Autodesk Fusion 360 part; units mm, degrees
(part 3 of 6)
  spline S106 degree 5 poles (-34.5944, 40.3997) (-34.5904, 40.3862) (-34.5823, 40.3594) (-34.5702, 40.3191) (-34.5538, 40.2655) (-34.5332, 40.1986) (-34.5123, 40.1318) (-34.4913, 40.0652) (-34.47, 39.9986) (-34.4485, 39.9322) (-34.4268, 39.8659) (-34.4049, 39.7998) (-34.3828, 39.7338) (-34.3605, 39.6679) (-34.338, 39.6021) (-34.3152, 39.5365) (-34.2923, 39.471) (-34.2691, 39.4056) (-34.2457, 39.3404) (-34.2221, 39.2753) (-34.1982, 39.2104) (-34.1742, 39.1456) (-34.1499, 39.0809) (-34.1254, 39.0164) (-34.1006, 38.9521) (-34.0756, 38.8878) (-34.0504, 38.8238) (-34.025, 38.7599) (-33.9993, 38.6961) (-33.9734, 38.6325) (-33.9473, 38.5691) (-33.9209, 38.5058) (-33.8943, 38.4427) (-33.8674, 38.3798) (-33.8403, 38.317) (-33.8129, 38.2544) (-33.7853, 38.1919) (-33.7574, 38.1297) (-33.7293, 38.0676) (-33.7009, 38.0057) (-33.6723, 37.944) (-33.6433, 37.8825) (-33.6142, 37.8211) (-33.589, 37.7688) (-33.5695, 37.7289) (-33.556, 37.7012) (-33.5483, 37.6857) (-33.5467, 37.6823) knots -1 -1 -1 -1 -1 -1 -0.985714 -0.971429 -0.957143 -0.942857 -0.928571 -0.914286 -0.9 -0.885714 -0.871429 -0.857143 -0.842857 -0.828571 -0.814286 -0.8 -0.785714 -0.771429 -0.757143 -0.742857 -0.728571 -0.714286 -0.7 -0.685714 -0.671429 -0.657143 -0.642857 -0.628571 -0.614286 -0.6 -0.585714 -0.571429 -0.557143 -0.542857 -0.528571 -0.514286 -0.5 -0.485714 -0.471429 -0.457143 -0.442857 -0.428571 -0.414286 -0.4 -0.396066 -0.396066 -0.396066 -0.396066 -0.396066 -0.396066
  spline S107 degree 3 poles (-33.6592, 37.0911) (-33.611, 37.1348) (-33.5718, 37.1876) (-33.5158, 37.3052) (-33.4995, 37.3688) (-33.4936, 37.4766) (-33.4967, 37.5194) (-33.5138, 37.6033) (-33.5278, 37.644) (-33.5467, 37.6823) knots 0 0 0 0 0.019532 0.019532 0.039064 0.039064 0.051902 0.051902 0.06474 0.06474 0.06474 0.06474
  arc A54 (-33.6592, 37.0911) -> (-34.0164, 36.7638) centre (0, 0) ccw
  spline S108 degree 3 poles (-34.6152, 36.7032) (-34.5595, 36.6695) (-34.4978, 36.6469) (-34.3691, 36.6267) (-34.3034, 36.6293) (-34.1985, 36.6543) (-34.1583, 36.6695) (-34.0828, 36.7098) (-34.0478, 36.7347) (-34.0164, 36.7638) knots 0 0 0 0 0.019532 0.019532 0.039064 0.039064 0.051902 0.051902 0.06474 0.06474 0.06474 0.06474
  spline S109 degree 5 poles (-34.6152, 36.7032) (-34.6184, 36.7052) (-34.6331, 36.7141) (-34.6595, 36.7301) (-34.6976, 36.7529) (-34.7475, 36.7826) (-34.8061, 36.817) (-34.8649, 36.8512) (-34.9239, 36.8851) (-34.983, 36.9188) (-35.0424, 36.9522) (-35.102, 36.9854) (-35.1618, 37.0183) (-35.2218, 37.0511) (-35.282, 37.0835) (-35.3423, 37.1158) (-35.4029, 37.1478) (-35.4636, 37.1796) (-35.5245, 37.2112) (-35.5856, 37.2425) (-35.6469, 37.2737) (-35.7084, 37.3046) (-35.77, 37.3353) (-35.8318, 37.3658) (-35.8937, 37.396) (-35.9559, 37.4261) (-36.0181, 37.4559) (-36.0806, 37.4855) (-36.1432, 37.5149) (-36.206, 37.5441) (-36.2689, 37.5731) (-36.332, 37.6019) (-36.3952, 37.6305) (-36.4586, 37.6589) (-36.5222, 37.6871) (-36.5859, 37.715) (-36.6497, 37.7428) (-36.7137, 37.7704) (-36.7779, 37.7978) (-36.8422, 37.8249) (-36.9066, 37.8519) (-36.9711, 37.8787) (-37.0359, 37.9053) (-37.1007, 37.9317) (-37.1527, 37.9527) (-37.1917, 37.9683) (-37.2178, 37.9787) (-37.2309, 37.9839) knots 0.396066 0.396066 0.396066 0.396066 0.396066 0.396066 0.4 0.414286 0.428571 0.442857 0.457143 0.471429 0.485714 0.5 0.514286 0.528571 0.542857 0.557143 0.571429 0.585714 0.6 0.614286 0.628571 0.642857 0.657143 0.671429 0.685714 0.7 0.714286 0.728571 0.742857 0.757143 0.771429 0.785714 0.8 0.814286 0.828571 0.842857 0.857143 0.871429 0.885714 0.9 0.914286 0.928571 0.942857 0.957143 0.971429 0.985714 1 1 1 1 1 1
  arc A55 (-37.2309, 37.9839) -> (-37.9839, 37.2309) centre (0, 0) ccw
  spline S110 degree 5 poles (-37.9839, 37.2309) (-37.9787, 37.2178) (-37.9683, 37.1917) (-37.9527, 37.1527) (-37.9317, 37.1007) (-37.9053, 37.0359) (-37.8787, 36.9711) (-37.8519, 36.9066) (-37.8249, 36.8422) (-37.7978, 36.7779) (-37.7704, 36.7137) (-37.7428, 36.6497) (-37.715, 36.5859) (-37.6871, 36.5222) (-37.6589, 36.4586) (-37.6305, 36.3952) (-37.6019, 36.332) (-37.5731, 36.2689) (-37.5441, 36.206) (-37.5149, 36.1432) (-37.4855, 36.0806) (-37.4559, 36.0181) (-37.4261, 35.9559) (-37.396, 35.8937) (-37.3658, 35.8318) (-37.3353, 35.77) (-37.3046, 35.7084) (-37.2737, 35.6469) (-37.2425, 35.5856) (-37.2112, 35.5245) (-37.1796, 35.4636) (-37.1478, 35.4029) (-37.1158, 35.3423) (-37.0835, 35.282) (-37.0511, 35.2218) (-37.0183, 35.1618) (-36.9854, 35.102) (-36.9522, 35.0424) (-36.9188, 34.983) (-36.8851, 34.9239) (-36.8512, 34.8649) (-36.817, 34.8061) (-36.7826, 34.7475) (-36.7529, 34.6976) (-36.7301, 34.6595) (-36.7141, 34.6331) (-36.7052, 34.6184) (-36.7032, 34.6152) knots -1 -1 -1 -1 -1 -1 -0.985714 -0.971429 -0.957143 -0.942857 -0.928571 -0.914286 -0.9 -0.885714 -0.871429 -0.857143 -0.842857 -0.828571 -0.814286 -0.8 -0.785714 -0.771429 -0.757143 -0.742857 -0.728571 -0.714286 -0.7 -0.685714 -0.671429 -0.657143 -0.642857 -0.628571 -0.614286 -0.6 -0.585714 -0.571429 -0.557143 -0.542857 -0.528571 -0.514286 -0.5 -0.485714 -0.471429 -0.457143 -0.442857 -0.428571 -0.414286 -0.4 -0.396066 -0.396066 -0.396066 -0.396066 -0.396066 -0.396066
  spline S111 degree 3 poles (-36.7638, 34.0164) (-36.7196, 34.0641) (-36.6851, 34.1201) (-36.6396, 34.2421) (-36.629, 34.307) (-36.6324, 34.4148) (-36.6393, 34.4572) (-36.6637, 34.5393) (-36.6811, 34.5786) (-36.7032, 34.6152) knots 0 0 0 0 0.019532 0.019532 0.039064 0.039064 0.051902 0.051902 0.06474 0.06474 0.06474 0.06474
  arc A56 (-36.7638, 34.0164) -> (-37.0911, 33.6592) centre (0, 0) ccw
  spline S112 degree 3 poles (-37.6823, 33.5467) (-37.6239, 33.5179) (-37.5605, 33.5008) (-37.4306, 33.4919) (-37.3654, 33.5002) (-37.263, 33.5342) (-37.2243, 33.5529) (-37.1526, 33.5996) (-37.1198, 33.6275) (-37.0911, 33.6592) knots 0 0 0 0 0.019532 0.019532 0.039064 0.039064 0.051902 0.051902 0.06474 0.06474 0.06474 0.06474
  spline S113 degree 5 poles (-37.6823, 33.5467) (-37.6857, 33.5483) (-37.7012, 33.556) (-37.7289, 33.5695) (-37.7688, 33.589) (-37.8211, 33.6142) (-37.8825, 33.6433) (-37.944, 33.6723) (-38.0057, 33.7009) (-38.0676, 33.7293) (-38.1297, 33.7574) (-38.1919, 33.7853) (-38.2544, 33.8129) (-38.317, 33.8403) (-38.3798, 33.8674) (-38.4427, 33.8943) (-38.5058, 33.9209) (-38.5691, 33.9473) (-38.6325, 33.9734) (-38.6961, 33.9993) (-38.7599, 34.025) (-38.8238, 34.0504) (-38.8878, 34.0756) (-38.9521, 34.1006) (-39.0164, 34.1254) (-39.0809, 34.1499) (-39.1456, 34.1742) (-39.2104, 34.1982) (-39.2753, 34.2221) (-39.3404, 34.2457) (-39.4056, 34.2691) (-39.471, 34.2923) (-39.5365, 34.3152) (-39.6021, 34.338) (-39.6679, 34.3605) (-39.7338, 34.3828) (-39.7998, 34.4049) (-39.8659, 34.4268) (-39.9322, 34.4485) (-39.9986, 34.47) (-40.0652, 34.4913) (-40.1318, 34.5123) (-40.1986, 34.5332) (-40.2655, 34.5538) (-40.3191, 34.5702) (-40.3594, 34.5823) (-40.3862, 34.5904) (-40.3997, 34.5944) knots 0.396066 0.396066 0.396066 0.396066 0.396066 0.396066 0.4 0.414286 0.428571 0.442857 0.457143 0.471429 0.485714 0.5 0.514286 0.528571 0.542857 0.557143 0.571429 0.585714 0.6 0.614286 0.628571 0.642857 0.657143 0.671429 0.685714 0.7 0.714286 0.728571 0.742857 0.757143 0.771429 0.785714 0.8 0.814286 0.828571 0.842857 0.857143 0.871429 0.885714 0.9 0.914286 0.928571 0.942857 0.957143 0.971429 0.985714 1 1 1 1 1 1
  arc A57 (-40.3997, 34.5944) -> (-41.0842, 33.7787) centre (0, 0) ccw
  spline S114 degree 5 poles (-41.0842, 33.7787) (-41.0779, 33.7661) (-41.0653, 33.7411) (-41.0463, 33.7035) (-41.0209, 33.6536) (-40.9889, 33.5913) (-40.9568, 33.5291) (-40.9245, 33.4671) (-40.892, 33.4053) (-40.8593, 33.3436) (-40.8265, 33.2821) (-40.7934, 33.2208) (-40.7602, 33.1596) (-40.7268, 33.0986) (-40.6931, 33.0377) (-40.6594, 32.977) (-40.6254, 32.9165) (-40.5912, 32.8562) (-40.5568, 32.796) (-40.5223, 32.736) (-40.4875, 32.6762) (-40.4525, 32.6166) (-40.4174, 32.5571) (-40.3821, 32.4979) (-40.3465, 32.4388) (-40.3108, 32.3799) (-40.2748, 32.3212) (-40.2387, 32.2626) (-40.2023, 32.2043) (-40.1658, 32.1462) (-40.129, 32.0883) (-40.092, 32.0305) (-40.0549, 31.973) (-40.0175, 31.9157) (-39.9799, 31.8586) (-39.942, 31.8016) (-39.904, 31.745) (-39.8657, 31.6885) (-39.8272, 31.6322) (-39.7885, 31.5762) (-39.7496, 31.5204) (-39.7104, 31.4648) (-39.6711, 31.4095) (-39.6372, 31.3624) (-39.6111, 31.3264) (-39.5929, 31.3015) (-39.5827, 31.2876) (-39.5805, 31.2845) knots -1 -1 -1 -1 -1 -1 -0.985714 -0.971429 -0.957143 -0.942857 -0.928571 -0.914286 -0.9 -0.885714 -0.871429 -0.857143 -0.842857 -0.828571 -0.814286 -0.8 -0.785714 -0.771429 -0.757143 -0.742857 -0.728571 -0.714286 -0.7 -0.685714 -0.671429 -0.657143 -0.642857 -0.628571 -0.614286 -0.6 -0.585714 -0.571429 -0.557143 -0.542857 -0.528571 -0.514286 -0.5 -0.485714 -0.471429 -0.457143 -0.442857 -0.428571 -0.414286 -0.4 -0.396066 -0.396066 -0.396066 -0.396066 -0.396066 -0.396066
  spline S115 degree 3 poles (-39.5886, 30.6827) (-39.5487, 30.7342) (-39.5193, 30.793) (-39.4846, 30.9185) (-39.4796, 30.984) (-39.4925, 31.0911) (-39.503, 31.1328) (-39.5344, 31.2124) (-39.5552, 31.25) (-39.5805, 31.2845) knots 0 0 0 0 0.019532 0.019532 0.039064 0.039064 0.051902 0.051902 0.06474 0.06474 0.06474 0.06474
  arc A58 (-39.5886, 30.6827) -> (-39.8835, 30.2984) centre (0, 0) ccw
  spline S116 degree 3 poles (-40.4627, 30.1348) (-40.402, 30.1112) (-40.3373, 30.0997) (-40.2071, 30.1022) (-40.1429, 30.1161) (-40.0439, 30.1589) (-40.0069, 30.1809) (-39.9396, 30.2337) (-39.9094, 30.2643) (-39.8835, 30.2984) knots 0 0 0 0 0.019532 0.019532 0.039064 0.039064 0.051902 0.051902 0.06474 0.06474 0.06474 0.06474
  spline S117 degree 5 poles (-40.4627, 30.1348) (-40.4662, 30.1361) (-40.4823, 30.1424) (-40.5111, 30.1535) (-40.5526, 30.1694) (-40.6069, 30.1899) (-40.6705, 30.2136) (-40.7343, 30.2371) (-40.7983, 30.2603) (-40.8624, 30.2831) (-40.9267, 30.3058) (-40.9912, 30.3281) (-41.0558, 30.3502) (-41.1205, 30.372) (-41.1855, 30.3935) (-41.2505, 30.4148) (-41.3157, 30.4358) (-41.381, 30.4566) (-41.4465, 30.4771) (-41.5121, 30.4974) (-41.5779, 30.5174) (-41.6437, 30.5372) (-41.7098, 30.5567) (-41.7759, 30.576) (-41.8422, 30.595) (-41.9086, 30.6138) (-41.9751, 30.6324) (-42.0417, 30.6507) (-42.1085, 30.6688) (-42.1754, 30.6866) (-42.2424, 30.7043) (-42.3095, 30.7217) (-42.3768, 30.7388) (-42.4441, 30.7558) (-42.5116, 30.7725) (-42.5792, 30.789) (-42.6469, 30.8052) (-42.7147, 30.8213) (-42.7826, 30.8371) (-42.8507, 30.8527) (-42.9188, 30.8681) (-42.987, 30.8833) (-43.0554, 30.8982) (-43.1238, 30.913) (-43.1787, 30.9246) (-43.2198, 30.9332) (-43.2473, 30.9389) (-43.2611, 30.9417) knots 0.396066 0.396066 0.396066 0.396066 0.396066 0.396066 0.4 0.414286 0.428571 0.442857 0.457143 0.471429 0.485714 0.5 0.514286 0.528571 0.542857 0.557143 0.571429 0.585714 0.6 0.614286 0.628571 0.642857 0.657143 0.671429 0.685714 0.7 0.714286 0.728571 0.742857 0.757143 0.771429 0.785714 0.8 0.814286 0.828571 0.842857 0.857143 0.871429 0.885714 0.9 0.914286 0.928571 0.942857 0.957143 0.971429 0.985714 1 1 1 1 1 1
  arc A59 (-43.2611, 30.9417) -> (-43.8719, 30.0694) centre (0, 0) ccw
  spline S118 degree 5 poles (-43.8719, 30.0694) (-43.8645, 30.0575) (-43.8498, 30.0336) (-43.8276, 29.9978) (-43.7979, 29.9503) (-43.7606, 29.891) (-43.7232, 29.8319) (-43.6856, 29.773) (-43.6479, 29.7142) (-43.6099, 29.6556) (-43.5718, 29.5972) (-43.5336, 29.539) (-43.4951, 29.4809) (-43.4565, 29.423) (-43.4177, 29.3654) (-43.3788, 29.3079) (-43.3396, 29.2505) (-43.3003, 29.1934) (-43.2608, 29.1365) (-43.2212, 29.0797) (-43.1813, 29.0232) (-43.1413, 28.9668) (-43.1011, 28.9106) (-43.0608, 28.8547) (-43.0202, 28.7989) (-42.9795, 28.7433) (-42.9385, 28.688) (-42.8974, 28.6328) (-42.8561, 28.5779) (-42.8146, 28.5232) (-42.773, 28.4687) (-42.7311, 28.4144) (-42.6891, 28.3603) (-42.6468, 28.3065) (-42.6044, 28.2528) (-42.5617, 28.1995) (-42.5189, 28.1463) (-42.4759, 28.0934) (-42.4326, 28.0407) (-42.3892, 27.9883) (-42.3455, 27.9361) (-42.3017, 27.8841) (-42.2576, 27.8324) (-42.2198, 27.7884) (-42.1906, 27.7549) (-42.1703, 27.7316) (-42.159, 27.7186) (-42.1565, 27.7158) knots -1 -1 -1 -1 -1 -1 -0.985714 -0.971429 -0.957143 -0.942857 -0.928571 -0.914286 -0.9 -0.885714 -0.871429 -0.857143 -0.842857 -0.828571 -0.814286 -0.8 -0.785714 -0.771429 -0.757143 -0.742857 -0.728571 -0.714286 -0.7 -0.685714 -0.671429 -0.657143 -0.642857 -0.628571 -0.614286 -0.6 -0.585714 -0.571429 -0.557143 -0.542857 -0.528571 -0.514286 -0.5 -0.485714 -0.471429 -0.457143 -0.442857 -0.428571 -0.414286 -0.4 -0.396066 -0.396066 -0.396066 -0.396066 -0.396066 -0.396066
  spline S119 degree 3 poles (-42.1121, 27.1156) (-42.0769, 27.1703) (-42.0527, 27.2314) (-42.029, 27.3595) (-42.0298, 27.4252) (-42.052, 27.5308) (-42.0661, 27.5714) (-42.1043, 27.648) (-42.1283, 27.6836) (-42.1565, 27.7158) knots 0 0 0 0 0.019532 0.019532 0.039064 0.039064 0.051902 0.051902 0.06474 0.06474 0.06474 0.06474
  arc A60 (-42.1121, 27.1156) -> (-42.3724, 26.707) centre (0, 0) ccw
  spline S120 degree 3 poles (-42.9352, 26.4935) (-42.8727, 26.4754) (-42.8072, 26.4695) (-42.6777, 26.4833) (-42.6149, 26.5028) (-42.52, 26.5541) (-42.4851, 26.5792) (-42.4226, 26.6377) (-42.3953, 26.6708) (-42.3724, 26.707) knots 0 0 0 0 0.019532 0.019532 0.039064 0.039064 0.051902 0.051902 0.06474 0.06474 0.06474 0.06474
  spline S121 degree 5 poles (-42.9352, 26.4935) (-42.9388, 26.4946) (-42.9554, 26.4994) (-42.985, 26.508) (-43.0277, 26.5202) (-43.0836, 26.5359) (-43.149, 26.554) (-43.2147, 26.5718) (-43.2804, 26.5893) (-43.3463, 26.6065) (-43.4123, 26.6234) (-43.4785, 26.6401) (-43.5448, 26.6564) (-43.6112, 26.6725) (-43.6777, 26.6883) (-43.7444, 26.7038) (-43.8111, 26.7191) (-43.878, 26.7341) (-43.945, 26.7488) (-44.0122, 26.7633) (-44.0794, 26.7775) (-44.1468, 26.7915) (-44.2142, 26.8052) (-44.2818, 26.8186) (-44.3495, 26.8318) (-44.4173, 26.8447) (-44.4852, 26.8574) (-44.5531, 26.8699) (-44.6212, 26.8821) (-44.6894, 26.894) (-44.7577, 26.9058) (-44.8261, 26.9172) (-44.8946, 26.9285) (-44.9632, 26.9395) (-45.0319, 26.9503) (-45.1006, 26.9608) (-45.1695, 26.9711) (-45.2384, 26.9812) (-45.3075, 26.991) (-45.3766, 27.0006) (-45.4458, 27.01) (-45.5151, 27.0192) (-45.5845, 27.0281) (-45.654, 27.0368) (-45.7096, 27.0436) (-45.7514, 27.0486) (-45.7793, 27.0519) (-45.7932, 27.0535) knots 0.396066 0.396066 0.396066 0.396066 0.396066 0.396066 0.4 0.414286 0.428571 0.442857 0.457143 0.471429 0.485714 0.5 0.514286 0.528571 0.542857 0.557143 0.571429 0.585714 0.6 0.614286 0.628571 0.642857 0.657143 0.671429 0.685714 0.7 0.714286 0.728571 0.742857 0.757143 0.771429 0.785714 0.8 0.814286 0.828571 0.842857 0.857143 0.871429 0.885714 0.9 0.914286 0.928571 0.942857 0.957143 0.971429 0.985714 1 1 1 1 1 1
  arc A61 (-45.7932, 27.0535) -> (-46.3256, 26.1313) centre (0, 0) ccw
  spline S122 degree 5 poles (-46.3256, 26.1313) (-46.3173, 26.12) (-46.3005, 26.0976) (-46.2753, 26.0639) (-46.2416, 26.0191) (-46.1993, 25.9633) (-46.1569, 25.9077) (-46.1143, 25.8522) (-46.0715, 25.797) (-46.0286, 25.7419) (-45.9856, 25.687) (-45.9424, 25.6324) (-45.899, 25.5779) (-45.8555, 25.5236) (-45.8119, 25.4695) (-45.768, 25.4156) (-45.7241, 25.3619) (-45.6799, 25.3084) (-45.6356, 25.2552) (-45.5912, 25.2021) (-45.5466, 25.1492) (-45.5018, 25.0966) (-45.4569, 25.0441) (-45.4118, 24.9919) (-45.3665, 24.9399) (-45.3211, 24.8881) (-45.2755, 24.8365) (-45.2297, 24.7851) (-45.1838, 24.734) (-45.1377, 24.6831) (-45.0914, 24.6324) (-45.045, 24.582) (-44.9984, 24.5318) (-44.9516, 24.4818) (-44.9046, 24.4321) (-44.8575, 24.3827) (-44.8102, 24.3334) (-44.7627, 24.2845) (-44.7151, 24.2357) (-44.6672, 24.1873) (-44.6192, 24.1391) (-44.571, 24.0912) (-44.5226, 24.0435) (-44.481, 24.003) (-44.4491, 23.9721) (-44.4268, 23.9507) (-44.4144, 23.9388) (-44.4117, 23.9362) knots -1 -1 -1 -1 -1 -1 -0.985714 -0.971429 -0.957143 -0.942857 -0.928571 -0.914286 -0.9 -0.885714 -0.871429 -0.857143 -0.842857 -0.828571 -0.814286 -0.8 -0.785714 -0.771429 -0.757143 -0.742857 -0.728571 -0.714286 -0.7 -0.685714 -0.671429 -0.657143 -0.642857 -0.628571 -0.614286 -0.6 -0.585714 -0.571429 -0.557143 -0.542857 -0.528571 -0.514286 -0.5 -0.485714 -0.471429 -0.457143 -0.442857 -0.428571 -0.414286 -0.4 -0.396066 -0.396066 -0.396066 -0.396066 -0.396066 -0.396066
  spline S123 degree 3 poles (-44.3152, 23.3421) (-44.2848, 23.3997) (-44.266, 23.4627) (-44.2536, 23.5923) (-44.2602, 23.6577) (-44.2914, 23.761) (-44.309, 23.8002) (-44.3538, 23.8731) (-44.3808, 23.9066) (-44.4117, 23.9362) knots 0 0 0 0 0.019532 0.019532 0.039064 0.039064 0.051902 0.051902 0.06474 0.06474 0.06474 0.06474
  arc A62 (-44.3152, 23.3421) -> (-44.5389, 22.9124) centre (0, 0) ccw
  spline S124 degree 3 poles (-45.0809, 22.6507) (-45.017, 22.638) (-44.9513, 22.6379) (-44.8235, 22.663) (-44.7626, 22.6878) (-44.6726, 22.7472) (-44.64, 22.7753) (-44.5828, 22.839) (-44.5585, 22.8743) (-44.5389, 22.9124) knots 0 0 0 0 0.019532 0.019532 0.039064 0.039064 0.051902 0.051902 0.06474 0.06474 0.06474 0.06474
  spline S125 degree 5 poles (-45.0809, 22.6507) (-45.0845, 22.6514) (-45.1015, 22.6548) (-45.1317, 22.6607) (-45.1754, 22.6692) (-45.2324, 22.68) (-45.2992, 22.6923) (-45.3661, 22.7043) (-45.4331, 22.716) (-45.5003, 22.7274) (-45.5675, 22.7385) (-45.6349, 22.7493) (-45.7023, 22.7598) (-45.7699, 22.77) (-45.8375, 22.78) (-45.9053, 22.7897) (-45.9731, 22.799) (-46.0411, 22.8081) (-46.1091, 22.817) (-46.1773, 22.8255) (-46.2455, 22.8338) (-46.3138, 22.8419) (-46.3822, 22.8496) (-46.4507, 22.8571) (-46.5193, 22.8644) (-46.5879, 22.8714) (-46.6566, 22.8781) (-46.7255, 22.8846) (-46.7944, 22.8908) (-46.8633, 22.8968) (-46.9324, 22.9025) (-47.0015, 22.908) (-47.0707, 22.9132) (-47.14, 22.9182) (-47.2094, 22.9229) (-47.2788, 22.9274) (-47.3483, 22.9317) (-47.4179, 22.9357) (-47.4875, 22.9395) (-47.5572, 22.9431) (-47.627, 22.9464) (-47.6968, 22.9495) (-47.7667, 22.9523) (-47.8367, 22.9549) (-47.8927, 22.9569) (-47.9347, 22.9582) (-47.9628, 22.959) (-47.9768, 22.9595) knots 0.396066 0.396066 0.396066 0.396066 0.396066 0.396066 0.4 0.414286 0.428571 0.442857 0.457143 0.471429 0.485714 0.5 0.514286 0.528571 0.542857 0.557143 0.571429 0.585714 0.6 0.614286 0.628571 0.642857 0.657143 0.671429 0.685714 0.7 0.714286 0.728571 0.742857 0.757143 0.771429 0.785714 0.8 0.814286 0.828571 0.842857 0.857143 0.871429 0.885714 0.9 0.914286 0.928571 0.942857 0.957143 0.971429 0.985714 1 1 1 1 1 1
  arc A63 (-47.9768, 22.9595) -> (-48.4269, 21.9943) centre (0, 0) ccw
  spline S126 degree 5 poles (-48.4269, 21.9943) (-48.4175, 21.9838) (-48.3989, 21.9629) (-48.3708, 21.9315) (-48.3333, 21.8899) (-48.2863, 21.8379) (-48.2392, 21.7862) (-48.192, 21.7347) (-48.1446, 21.6834) (-48.097, 21.6323) (-48.0494, 21.5814) (-48.0016, 21.5307) (-47.9536, 21.4802) (-47.9056, 21.4299) (-47.8574, 21.3798) (-47.809, 21.33) (-47.7605, 21.2803) (-47.7119, 21.2309) (-47.6631, 21.1817) (-47.6142, 21.1327) (-47.5651, 21.0839) (-47.5159, 21.0353) (-47.4666, 20.987) (-47.4171, 20.9389) (-47.3675, 20.891) (-47.3177, 20.8434) (-47.2678, 20.796) (-47.2178, 20.7488) (-47.1676, 20.7019) (-47.1172, 20.6552) (-47.0667, 20.6087) (-47.016, 20.5625) (-46.9652, 20.5166) (-46.9143, 20.4709) (-46.8632, 20.4255) (-46.8119, 20.3803) (-46.7605, 20.3354) (-46.7089, 20.2907) (-46.6572, 20.2463) (-46.6053, 20.2022) (-46.5533, 20.1584) (-46.501, 20.1149) (-46.4487, 20.0716) (-46.4038, 20.0349) (-46.3692, 20.0069) (-46.3452, 19.9875) (-46.3318, 19.9767) (-46.3288, 19.9744) knots -1 -1 -1 -1 -1 -1 -0.985714 -0.971429 -0.957143 -0.942857 -0.928571 -0.914286 -0.9 -0.885714 -0.871429 -0.857143 -0.842857 -0.828571 -0.814286 -0.8 -0.785714 -0.771429 -0.757143 -0.742857 -0.728571 -0.714286 -0.7 -0.685714 -0.671429 -0.657143 -0.642857 -0.628571 -0.614286 -0.6 -0.585714 -0.571429 -0.557143 -0.542857 -0.528571 -0.514286 -0.5 -0.485714 -0.471429 -0.457143 -0.442857 -0.428571 -0.414286 -0.4 -0.396066 -0.396066 -0.396066 -0.396066 -0.396066 -0.396066
  spline S127 degree 3 poles (-46.1809, 19.391) (-46.1557, 19.451) (-46.1425, 19.5154) (-46.1414, 19.6456) (-46.1536, 19.7102) (-46.1938, 19.8103) (-46.2147, 19.8478) (-46.2657, 19.9166) (-46.2955, 19.9476) (-46.3288, 19.9744) knots 0 0 0 0 0.019532 0.019532 0.039064 0.039064 0.051902 0.051902 0.06474 0.06474 0.06474 0.06474
  arc A64 (-46.1809, 19.391) -> (-46.3663, 18.9434) centre (0, 0) ccw
  spline S128 degree 3 poles (-46.8834, 18.6354) (-46.8187, 18.6284) (-46.7532, 18.634) (-46.6281, 18.6701) (-46.5697, 18.7002) (-46.4851, 18.7672) (-46.4551, 18.798) (-46.4037, 18.8664) (-46.3825, 18.9038) (-46.3663, 18.9434) knots 0 0 0 0 0.019532 0.019532 0.039064 0.039064 0.051902 0.051902 0.06474 0.06474 0.06474 0.06474
  spline S129 degree 5 poles (-46.8834, 18.6354) (-46.8872, 18.6358) (-46.9043, 18.6377) (-46.935, 18.641) (-46.9792, 18.6456) (-47.0369, 18.6514) (-47.1046, 18.6578) (-47.1723, 18.664) (-47.2401, 18.6698) (-47.3079, 18.6753) (-47.3759, 18.6805) (-47.4439, 18.6854) (-47.5121, 18.69) (-47.5802, 18.6943) (-47.6485, 18.6983) (-47.7169, 18.702) (-47.7853, 18.7055) (-47.8537, 18.7086) (-47.9223, 18.7115) (-47.9909, 18.7141) (-48.0596, 18.7164) (-48.1284, 18.7184) (-48.1972, 18.7202) (-48.2661, 18.7217) (-48.335, 18.723) (-48.404, 18.7239) (-48.4731, 18.7246) (-48.5422, 18.7251) (-48.6114, 18.7253) (-48.6806, 18.7252) (-48.7499, 18.7249) (-48.8192, 18.7243) (-48.8886, 18.7235) (-48.9581, 18.7224) (-49.0276, 18.7211) (-49.0971, 18.7196) (-49.1667, 18.7177) (-49.2364, 18.7157) (-49.3061, 18.7134) (-49.3758, 18.7109) (-49.4456, 18.7081) (-49.5155, 18.7051) (-49.5854, 18.7018) (-49.6553, 18.6984) (-49.7113, 18.6954) (-49.7533, 18.6931) (-49.7813, 18.6914) (-49.7953, 18.6906) knots 0.396066 0.396066 0.396066 0.396066 0.396066 0.396066 0.4 0.414286 0.428571 0.442857 0.457143 0.471429 0.485714 0.5 0.514286 0.528571 0.542857 0.557143 0.571429 0.585714 0.6 0.614286 0.628571 0.642857 0.657143 0.671429 0.685714 0.7 0.714286 0.728571 0.742857 0.757143 0.771429 0.785714 0.8 0.814286 0.828571 0.842857 0.857143 0.871429 0.885714 0.9 0.914286 0.928571 0.942857 0.957143 0.971429 0.985714 1 1 1 1 1 1
  arc A65 (-49.7953, 18.6906) -> (-50.1595, 17.6899) centre (0, 0) ccw
  spline S130 degree 5 poles (-50.1595, 17.6899) (-50.1493, 17.6803) (-50.1289, 17.6611) (-50.0982, 17.6323) (-50.0572, 17.594) (-50.0059, 17.5464) (-49.9544, 17.499) (-49.9029, 17.4518) (-49.8512, 17.4048) (-49.7994, 17.358) (-49.7475, 17.3115) (-49.6954, 17.2651) (-49.6433, 17.219) (-49.591, 17.1731) (-49.5386, 17.1274) (-49.4861, 17.082) (-49.4335, 17.0367) (-49.3807, 16.9917) (-49.3278, 16.9469) (-49.2748, 16.9024) (-49.2217, 16.8581) (-49.1685, 16.814) (-49.1151, 16.7701) (-49.0616, 16.7265) (-49.008, 16.6832) (-48.9543, 16.64) (-48.9004, 16.5972) (-48.8465, 16.5545) (-48.7924, 16.5122) (-48.7381, 16.47) (-48.6838, 16.4282) (-48.6293, 16.3866) (-48.5747, 16.3452) (-48.5199, 16.3041) (-48.465, 16.2633) (-48.41, 16.2228) (-48.3549, 16.1825) (-48.2996, 16.1426) (-48.2442, 16.1029) (-48.1887, 16.0634) (-48.133, 16.0243) (-48.0772, 15.9855) (-48.0213, 15.947) (-47.9733, 15.9143) (-47.9365, 15.8894) (-47.9109, 15.8722) (-47.8965, 15.8626) (-47.8934, 15.8605) knots -1 -1 -1 -1 -1 -1 -0.985714 -0.971429 -0.957143 -0.942857 -0.928571 -0.914286 -0.9 -0.885714 -0.871429 -0.857143 -0.842857 -0.828571 -0.814286 -0.8 -0.785714 -0.771429 -0.757143 -0.742857 -0.728571 -0.714286 -0.7 -0.685714 -0.671429 -0.657143 -0.642857 -0.628571 -0.614286 -0.6 -0.585714 -0.571429 -0.557143 -0.542857 -0.528571 -0.514286 -0.5 -0.485714 -0.471429 -0.457143 -0.442857 -0.428571 -0.414286 -0.4 -0.396066 -0.396066 -0.396066 -0.396066 -0.396066 -0.396066
  spline S131 degree 3 poles (-47.6952, 15.2922) (-47.6754, 15.3542) (-47.6678, 15.4195) (-47.6781, 15.5493) (-47.6959, 15.6126) (-47.7446, 15.7089) (-47.7687, 15.7444) (-47.8255, 15.8085) (-47.8579, 15.8367) (-47.8934, 15.8605) knots 0 0 0 0 0.019532 0.019532 0.039064 0.039064 0.051902 0.051902 0.06474 0.06474 0.06474 0.06474
  arc A66 (-47.6952, 15.2922) -> (-47.8409, 14.8302) centre (0, 0) ccw
  spline S132 degree 3 poles (-48.3292, 14.4784) (-48.2641, 14.477) (-48.1994, 14.4883) (-48.0779, 14.5351) (-48.0223, 14.5702) (-47.9439, 14.6443) (-47.9167, 14.6776) (-47.8715, 14.7502) (-47.8536, 14.7893) (-47.8409, 14.8302) knots 0 0 0 0 0.019532 0.019532 0.039064 0.039064 0.051902 0.051902 0.06474 0.06474 0.06474 0.06474
  spline S133 degree 5 poles (-48.3292, 14.4784) (-48.333, 14.4784) (-48.3502, 14.4788) (-48.3811, 14.4794) (-48.4255, 14.4801) (-48.4835, 14.4809) (-48.5515, 14.4814) (-48.6194, 14.4816) (-48.6875, 14.4815) (-48.7556, 14.4811) (-48.8237, 14.4803) (-48.8919, 14.4793) (-48.9602, 14.4779) (-49.0285, 14.4763) (-49.0969, 14.4743) (-49.1653, 14.4721) (-49.2337, 14.4695) (-49.3022, 14.4667) (-49.3708, 14.4636) (-49.4393, 14.4602) (-49.508, 14.4565) (-49.5766, 14.4525) (-49.6453, 14.4483) (-49.7141, 14.4438) (-49.7829, 14.439) (-49.8517, 14.434) (-49.9206, 14.4287) (-49.9895, 14.4231) (-50.0584, 14.4173) (-50.1274, 14.4112) (-50.1964, 14.4048) (-50.2654, 14.3982) (-50.3345, 14.3913) (-50.4035, 14.3842) (-50.4727, 14.3768) (-50.5418, 14.3692) (-50.611, 14.3614) (-50.6802, 14.3532) (-50.7494, 14.3449) (-50.8187, 14.3363) (-50.888, 14.3274) (-50.9573, 14.3183) (-51.0266, 14.309) (-51.096, 14.2995) (-51.1515, 14.2916) (-51.1931, 14.2856) (-51.2209, 14.2816) (-51.2348, 14.2796) knots 0.396066 0.396066 0.396066 0.396066 0.396066 0.396066 0.4 0.414286 0.428571 0.442857 0.457143 0.471429 0.485714 0.5 0.514286 0.528571 0.542857 0.557143 0.571429 0.585714 0.6 0.614286 0.628571 0.642857 0.657143 0.671429 0.685714 0.7 0.714286 0.728571 0.742857 0.757143 0.771429 0.785714 0.8 0.814286 0.828571 0.842857 0.857143 0.871429 0.885714 0.9 0.914286 0.928571 0.942857 0.957143 0.971429 0.985714 1 1 1 1 1 1
  arc A67 (-51.2348, 14.2796) -> (-51.5104, 13.2509) centre (0, 0) ccw
  spline S134 degree 5 poles (-51.5104, 13.2509) (-51.4994, 13.2422) (-51.4774, 13.2248) (-51.4443, 13.1988) (-51.4002, 13.1643) (-51.3449, 13.1213) (-51.2895, 13.0786) (-51.234, 13.0361) (-51.1784, 12.9938) (-51.1228, 12.9517) (-51.067, 12.9098) (-51.0111, 12.8682) (-50.9551, 12.8268) (-50.899, 12.7856) (-50.8429, 12.7447) (-50.7866, 12.704) (-50.7302, 12.6635) (-50.6737, 12.6232) (-50.6172, 12.5832) (-50.5605, 12.5435) (-50.5037, 12.504) (-50.4468, 12.4647) (-50.3898, 12.4257) (-50.3328, 12.3869) (-50.2756, 12.3483) (-50.2183, 12.3101) (-50.1609, 12.272) (-50.1034, 12.2343) (-50.0458, 12.1968) (-49.9881, 12.1596) (-49.9303, 12.1226) (-49.8724, 12.0859) (-49.8144, 12.0495) (-49.7563, 12.0133) (-49.6981, 11.9774) (-49.6397, 11.9419) (-49.5813, 11.9065) (-49.5228, 11.8715) (-49.4641, 11.8368) (-49.4053, 11.8024) (-49.3465, 11.7683) (-49.2875, 11.7345) (-49.2284, 11.701) (-49.1778, 11.6726) (-49.139, 11.651) (-49.1119, 11.6361) (-49.0968, 11.6278) (-49.0935, 11.626) knots -1 -1 -1 -1 -1 -1 -0.985714 -0.971429 -0.957143 -0.942857 -0.928571 -0.914286 -0.9 -0.885714 -0.871429 -0.857143 -0.842857 -0.828571 -0.814286 -0.8 -0.785714 -0.771429 -0.757143 -0.742857 -0.728571 -0.714286 -0.7 -0.685714 -0.671429 -0.657143 -0.642857 -0.628571 -0.614286 -0.6 -0.585714 -0.571429 -0.557143 -0.542857 -0.528571 -0.514286 -0.5 -0.485714 -0.471429 -0.457143 -0.442857 -0.428571 -0.414286 -0.4 -0.396066 -0.396066 -0.396066 -0.396066 -0.396066 -0.396066
  spline S135 degree 3 poles (-48.8466, 11.0771) (-48.8322, 11.1406) (-48.8303, 11.2063) (-48.8519, 11.3347) (-48.8751, 11.3962) (-48.932, 11.4879) (-48.9592, 11.5212) (-49.0213, 11.5801) (-49.056, 11.6054) (-49.0935, 11.626) knots 0 0 0 0 0.019532 0.019532 0.039064 0.039064 0.051902 0.051902 0.06474 0.06474 0.06474 0.06474
  arc A68 (-48.8466, 11.0771) -> (-48.9514, 10.6042) centre (0, 0) ccw
  spline S136 degree 3 poles (-49.4072, 10.2111) (-49.3422, 10.2154) (-49.2787, 10.2323) (-49.1618, 10.2896) (-49.1094, 10.3293) (-49.0378, 10.41) (-49.0136, 10.4455) (-48.9749, 10.5218) (-48.9605, 10.5623) (-48.9514, 10.6042) knots 0 0 0 0 0.019532 0.019532 0.039064 0.039064 0.051902 0.051902 0.06474 0.06474 0.06474 0.06474
  spline S137 degree 5 poles (-49.4072, 10.2111) (-49.4109, 10.2109) (-49.4282, 10.2097) (-49.4589, 10.2076) (-49.5033, 10.2045) (-49.5611, 10.2002) (-49.6288, 10.1948) (-49.6966, 10.189) (-49.7644, 10.183) (-49.8322, 10.1766) (-49.9, 10.17) (-49.9678, 10.163) (-50.0357, 10.1557) (-50.1036, 10.1481) (-50.1715, 10.1402) (-50.2395, 10.132) (-50.3075, 10.1235) (-50.3755, 10.1147) (-50.4435, 10.1056) (-50.5115, 10.0962) (-50.5795, 10.0866) (-50.6476, 10.0767) (-50.7157, 10.0665) (-50.7838, 10.056) (-50.8519, 10.0452) (-50.92, 10.0342) (-50.9881, 10.0229) (-51.0563, 10.0114) (-51.1245, 9.9995) (-51.1926, 9.9874) (-51.2608, 9.9751) (-51.329, 9.9625) (-51.3972, 9.9496) (-51.4654, 9.9365) (-51.5336, 9.9232) (-51.6019, 9.9095) (-51.6701, 9.8957) (-51.7383, 9.8816) (-51.8066, 9.8672) (-51.8748, 9.8526) (-51.9431, 9.8377) (-52.0113, 9.8226) (-52.0796, 9.8073) (-52.1478, 9.7917) (-52.2025, 9.7791) (-52.2434, 9.7695) (-52.2707, 9.7631) (-52.2844, 9.7598) knots 0.396066 0.396066 0.396066 0.396066 0.396066 0.396066 0.4 0.414286 0.428571 0.442857 0.457143 0.471429 0.485714 0.5 0.514286 0.528571 0.542857 0.557143 0.571429 0.585714 0.6 0.614286 0.628571 0.642857 0.657143 0.671429 0.685714 0.7 0.714286 0.728571 0.742857 0.757143 0.771429 0.785714 0.8 0.814286 0.828571 0.842857 0.857143 0.871429 0.885714 0.9 0.914286 0.928571 0.942857 0.957143 0.971429 0.985714 1 1 1 1 1 1
  arc A69 (-52.2844, 9.7598) -> (-52.4693, 8.7111) centre (0, 0) ccw
  spline S138 degree 5 poles (-52.4693, 8.7111) (-52.4576, 8.7034) (-52.4341, 8.688) (-52.3989, 8.665) (-52.3519, 8.6344) (-52.2931, 8.5964) (-52.2342, 8.5587) (-52.1752, 8.5211) (-52.1162, 8.4838) (-52.057, 8.4468) (-51.9978, 8.4099) (-51.9385, 8.3733) (-51.8791, 8.337) (-51.8197, 8.3008) (-51.7602, 8.2649) (-51.7006, 8.2293) (-51.6409, 8.1939) (-51.5811, 8.1587) (-51.5212, 8.1238) (-51.4613, 8.0891) (-51.4013, 8.0547) (-51.3412, 8.0205) (-51.2811, 7.9866) (-51.2208, 7.9529) (-51.1605, 7.9196) (-51.1001, 7.8864) (-51.0396, 7.8535) (-50.979, 7.8209) (-50.9184, 7.7886) (-50.8577, 7.7565) (-50.7969, 7.7247) (-50.736, 7.6932) (-50.675, 7.662) (-50.614, 7.6311) (-50.5528, 7.6004) (-50.4916, 7.57) (-50.4303, 7.5399) (-50.369, 7.5102) (-50.3075, 7.4807) (-50.246, 7.4515) (-50.1844, 7.4227) (-50.1227, 7.3941) (-50.0609, 7.3659) (-50.008, 7.342) (-49.9674, 7.3239) (-49.9392, 7.3114) (-49.9234, 7.3045) (-49.92, 7.303) knots -1 -1 -1 -1 -1 -1 -0.985714 -0.971429 -0.957143 -0.942857 -0.928571 -0.914286 -0.9 -0.885714 -0.871429 -0.857143 -0.842857 -0.828571 -0.814286 -0.8 -0.785714 -0.771429 -0.757143 -0.742857 -0.728571 -0.714286 -0.7 -0.685714 -0.671429 -0.657143 -0.642857 -0.628571 -0.614286 -0.6 -0.585714 -0.571429 -0.557143 -0.542857 -0.528571 -0.514286 -0.5 -0.485714 -0.471429 -0.457143 -0.442857 -0.428571 -0.414286 -0.4 -0.396066 -0.396066 -0.396066 -0.396066 -0.396066 -0.396066
  spline S139 degree 3 poles (-49.6261, 6.7777) (-49.6173, 6.8422) (-49.6212, 6.9078) (-49.6539, 7.0339) (-49.6824, 7.0931) (-49.7471, 7.1795) (-49.777, 7.2103) (-49.844, 7.2635) (-49.8808, 7.2857) (-49.92, 7.303) knots 0 0 0 0 0.019532 0.019532 0.039064 0.039064 0.051902 0.051902 0.06474 0.06474 0.06474 0.06474
  arc A70 (-49.6261, 6.7777) -> (-49.6893, 6.2974) centre (0, 0) ccw
  spline S140 degree 3 poles (-50.1091, 5.8661) (-50.0448, 5.876) (-49.983, 5.8984) (-49.8715, 5.9657) (-49.8228, 6.0099) (-49.7585, 6.0965) (-49.7375, 6.134) (-49.7055, 6.2134) (-49.6947, 6.255) (-49.6893, 6.2974) knots 0 0 0 0 0.019532 0.019532 0.039064 0.039064 0.051902 0.051902 0.06474 0.06474 0.06474 0.06474
  spline S141 degree 5 poles (-50.1091, 5.8661) (-50.1128, 5.8656) (-50.1299, 5.8629) (-50.1604, 5.8581) (-50.2043, 5.8512) (-50.2615, 5.8418) (-50.3285, 5.8305) (-50.3955, 5.8189) (-50.4625, 5.807) (-50.5295, 5.7947) (-50.5965, 5.7822) (-50.6635, 5.7693) (-50.7304, 5.7561) (-50.7974, 5.7426) (-50.8644, 5.7288) (-50.9314, 5.7147) (-50.9984, 5.7003) (-51.0653, 5.6857) (-51.1323, 5.6707) (-51.1992, 5.6554) (-51.2662, 5.6399) (-51.3331, 5.6241) (-51.4, 5.608) (-51.467, 5.5916) (-51.5339, 5.575) (-51.6008, 5.558) (-51.6677, 5.5409) (-51.7346, 5.5234) (-51.8014, 5.5057) (-51.8683, 5.4877) (-51.9351, 5.4695) (-52.002, 5.451) (-52.0688, 5.4322) (-52.1356, 5.4132) (-52.2024, 5.3939) (-52.2692, 5.3744) (-52.3359, 5.3547) (-52.4027, 5.3347) (-52.4694, 5.3144) (-52.5361, 5.2939) (-52.6028, 5.2732) (-52.6695, 5.2522) (-52.7362, 5.231) (-52.8028, 5.2095) (-52.8561, 5.1921) (-52.8961, 5.179) (-52.9227, 5.1702) (-52.936, 5.1658) knots 0.396066 0.396066 0.396066 0.396066 0.396066 0.396066 0.4 0.414286 0.428571 0.442857 0.457143 0.471429 0.485714 0.5 0.514286 0.528571 0.542857 0.557143 0.571429 0.585714 0.6 0.614286 0.628571 0.642857 0.657143 0.671429 0.685714 0.7 0.714286 0.728571 0.742857 0.757143 0.771429 0.785714 0.8 0.814286 0.828571 0.842857 0.857143 0.871429 0.885714 0.9 0.914286 0.928571 0.942857 0.957143 0.971429 0.985714 1 1 1 1 1 1
  arc A71 (-52.936, 5.1658) -> (-53.0289, 4.1049) centre (0, 0) ccw
  spline S142 degree 5 poles (-53.0289, 4.1049) (-53.0165, 4.0983) (-52.9918, 4.085) (-52.9547, 4.0651) (-52.9052, 4.0388) (-52.8433, 4.0061) (-52.7814, 3.9736) (-52.7193, 3.9413) (-52.6573, 3.9093) (-52.5951, 3.8776) (-52.5329, 3.846) (-52.4707, 3.8147) (-52.4083, 3.7837) (-52.346, 3.7529) (-52.2835, 3.7223) (-52.221, 3.692) (-52.1585, 3.6619) (-52.0959, 3.6321) (-52.0332, 3.6025) (-51.9705, 3.5732) (-51.9077, 3.5441) (-51.8449, 3.5153) (-51.782, 3.4868) (-51.719, 3.4585) (-51.656, 3.4305) (-51.593, 3.4027) (-51.5299, 3.3753) (-51.4667, 3.3481) (-51.4035, 3.3211) (-51.3402, 3.2945) (-51.2768, 3.2681) (-51.2134, 3.242) (-51.15, 3.2162) (-51.0865, 3.1907) (-51.0229, 3.1655) (-50.9593, 3.1406) (-50.8956, 3.116) (-50.8319, 3.0916) (-50.7681, 3.0676) (-50.7042, 3.0439) (-50.6403, 3.0206) (-50.5764, 2.9975) (-50.5124, 2.9748) (-50.4576, 2.9556) (-50.4156, 2.9411) (-50.3864, 2.9311) (-50.37, 2.9256) (-50.3665, 2.9244) knots -1 -1 -1 -1 -1 -1 -0.985714 -0.971429 -0.957143 -0.942857 -0.928571 -0.914286 -0.9 -0.885714 -0.871429 -0.857143 -0.842857 -0.828571 -0.814286 -0.8 -0.785714 -0.771429 -0.757143 -0.742857 -0.728571 -0.714286 -0.7 -0.685714 -0.671429 -0.657143 -0.642857 -0.628571 -0.614286 -0.6 -0.585714 -0.571429 -0.557143 -0.542857 -0.528571 -0.514286 -0.5 -0.485714 -0.471429 -0.457143 -0.442857 -0.428571 -0.414286 -0.4 -0.396066 -0.396066 -0.396066 -0.396066 -0.396066 -0.396066
  spline S143 degree 3 poles (-50.028, 2.4267) (-50.0248, 2.4918) (-50.0344, 2.5568) (-50.078, 2.6795) (-50.1115, 2.736) (-50.1835, 2.8164) (-50.216, 2.8445) (-50.2874, 2.8917) (-50.326, 2.9106) (-50.3665, 2.9244) knots 0 0 0 0 0.019532 0.019532 0.039064 0.039064 0.051902 0.051902 0.06474 0.06474 0.06474 0.06474
  arc A72 (-50.028, 2.4267) -> (-50.0491, 1.9427) centre (0, 0) ccw
  spline S144 degree 3 poles (-50.4297, 1.4765) (-50.3665, 1.492) (-50.3069, 1.5197) (-50.2017, 1.5964) (-50.157, 1.6446) (-50.1005, 1.7365) (-50.0828, 1.7757) (-50.0579, 1.8576) (-50.0508, 1.9) (-50.0491, 1.9427) knots 0 0 0 0 0.019532 0.019532 0.039064 0.039064 0.051902 0.051902 0.06474 0.06474 0.06474 0.06474
  spline S145 degree 5 poles (-50.4297, 1.4765) (-50.4334, 1.4756) (-50.4501, 1.4715) (-50.4801, 1.4641) (-50.5232, 1.4533) (-50.5794, 1.439) (-50.6452, 1.4219) (-50.7109, 1.4045) (-50.7766, 1.3868) (-50.8423, 1.3688) (-50.9079, 1.3504) (-50.9735, 1.3317) (-51.0391, 1.3128) (-51.1046, 1.2935) (-51.1702, 1.2739) (-51.2356, 1.254) (-51.3011, 1.2339) (-51.3665, 1.2134) (-51.4319, 1.1926) (-51.4973, 1.1716) (-51.5626, 1.1503) (-51.6279, 1.1287) (-51.6932, 1.1068) (-51.7585, 1.0847) (-51.8237, 1.0623) (-51.8888, 1.0396) (-51.954, 1.0166) (-52.0191, 0.9934) (-52.0842, 0.9699) (-52.1492, 0.9462) (-52.2142, 0.9222) (-52.2792, 0.898) (-52.3441, 0.8734) (-52.409, 0.8487) (-52.4739, 0.8237) (-52.5387, 0.7984) (-52.6035, 0.7729) (-52.6682, 0.7472) (-52.7329, 0.7212) (-52.7976, 0.6949) (-52.8622, 0.6685) (-52.9268, 0.6417) (-52.9914, 0.6148) (-53.0559, 0.5876) (-53.1075, 0.5657) (-53.1462, 0.5491) (-53.1719, 0.538) (-53.1848, 0.5325) knots 0.396066 0.396066 0.396066 0.396066 0.396066 0.396066 0.4 0.414286 0.428571 0.442857 0.457143 0.471429 0.485714 0.5 0.514286 0.528571 0.542857 0.557143 0.571429 0.585714 0.6 0.614286 0.628571 0.642857 0.657143 0.671429 0.685714 0.7 0.714286 0.728571 0.742857 0.757143 0.771429 0.785714 0.8 0.814286 0.828571 0.842857 0.857143 0.871429 0.885714 0.9 0.914286 0.928571 0.942857 0.957143 0.971429 0.985714 1 1 1 1 1 1
  arc A73 (-53.1848, 0.5325) -> (-53.1848, -0.5325) centre (0, 0) ccw
  spline S146 degree 5 poles (-53.1848, -0.5325) (-53.1719, -0.538) (-53.1462, -0.5491) (-53.1075, -0.5657) (-53.0559, -0.5876) (-52.9914, -0.6148) (-52.9268, -0.6417) (-52.8622, -0.6685) (-52.7976, -0.6949) (-52.7329, -0.7212) (-52.6682, -0.7472) (-52.6035, -0.7729) (-52.5387, -0.7984) (-52.4739, -0.8237) (-52.409, -0.8487) (-52.3441, -0.8734) (-52.2792, -0.898) (-52.2142, -0.9222) (-52.1492, -0.9462) (-52.0842, -0.9699) (-52.0191, -0.9934) (-51.954, -1.0166) (-51.8888, -1.0396) (-51.8237, -1.0623) (-51.7585, -1.0847) (-51.6932, -1.1068) (-51.6279, -1.1287) (-51.5626, -1.1503) (-51.4973, -1.1716) (-51.4319, -1.1926) (-51.3665, -1.2134) (-51.3011, -1.2339) (-51.2356, -1.254) (-51.1702, -1.2739) (-51.1046, -1.2935) (-51.0391, -1.3128) (-50.9735, -1.3317) (-50.9079, -1.3504) (-50.8423, -1.3688) (-50.7766, -1.3868) (-50.7109, -1.4045) (-50.6452, -1.4219) (-50.5794, -1.439) (-50.5232, -1.4533) (-50.4801, -1.4641) (-50.4501, -1.4715) (-50.4334, -1.4756) (-50.4297, -1.4765) knots -1 -1 -1 -1 -1 -1 -0.985714 -0.971429 -0.957143 -0.942857 -0.928571 -0.914286 -0.9 -0.885714 -0.871429 -0.857143 -0.842857 -0.828571 -0.814286 -0.8 -0.785714 -0.771429 -0.757143 -0.742857 -0.728571 -0.714286 -0.7 -0.685714 -0.671429 -0.657143 -0.642857 -0.628571 -0.614286 -0.6 -0.585714 -0.571429 -0.557143 -0.542857 -0.528571 -0.514286 -0.5 -0.485714 -0.471429 -0.457143 -0.442857 -0.428571 -0.414286 -0.4 -0.396066 -0.396066 -0.396066 -0.396066 -0.396066 -0.396066
  spline S147 degree 3 poles (-50.0491, -1.9427) (-50.0516, -1.8777) (-50.0669, -1.8137) (-50.1209, -1.6953) (-50.1593, -1.6419) (-50.238, -1.5681) (-50.2728, -1.543) (-50.3481, -1.5022) (-50.3882, -1.4867) (-50.4297, -1.4765) knots 0 0 0 0 0.019532 0.019532 0.039064 0.039064 0.051902 0.051902 0.06474 0.06474 0.06474 0.06474
  arc A74 (-50.0491, -1.9427) -> (-50.028, -2.4267) centre (0, 0) ccw
  spline S148 degree 3 poles (-50.3665, -2.9244) (-50.3049, -2.9034) (-50.2479, -2.8706) (-50.1498, -2.785) (-50.1095, -2.7331) (-50.0612, -2.6366) (-50.047, -2.596) (-50.0293, -2.5123) (-50.0259, -2.4695) (-50.028, -2.4267) knots 0 0 0 0 0.019532 0.019532 0.039064 0.039064 0.051902 0.051902 0.06474 0.06474 0.06474 0.06474
  spline S149 degree 5 poles (-50.3665, -2.9244) (-50.37, -2.9256) (-50.3864, -2.9311) (-50.4156, -2.9411) (-50.4576, -2.9556) (-50.5124, -2.9748) (-50.5764, -2.9975) (-50.6403, -3.0206) (-50.7042, -3.0439) (-50.7681, -3.0676) (-50.8319, -3.0916) (-50.8956, -3.116) (-50.9593, -3.1406) (-51.0229, -3.1655) (-51.0865, -3.1907) (-51.15, -3.2162) (-51.2134, -3.242) (-51.2768, -3.2681) (-51.3402, -3.2945) (-51.4035, -3.3211) (-51.4667, -3.3481) (-51.5299, -3.3753) (-51.593, -3.4027) (-51.656, -3.4305) (-51.719, -3.4585) (-51.782, -3.4868) (-51.8449, -3.5153) (-51.9077, -3.5441) (-51.9705, -3.5732) (-52.0332, -3.6025) (-52.0959, -3.6321) (-52.1585, -3.6619) (-52.221, -3.692) (-52.2835, -3.7223) (-52.346, -3.7529) (-52.4083, -3.7837) (-52.4707, -3.8147) (-52.5329, -3.846) (-52.5951, -3.8776) (-52.6573, -3.9093) (-52.7193, -3.9413) (-52.7814, -3.9736) (-52.8433, -4.0061) (-52.9052, -4.0388) (-52.9547, -4.0651) (-52.9918, -4.085) (-53.0165, -4.0983) (-53.0289, -4.1049) knots 0.396066 0.396066 0.396066 0.396066 0.396066 0.396066 0.4 0.414286 0.428571 0.442857 0.457143 0.471429 0.485714 0.5 0.514286 0.528571 0.542857 0.557143 0.571429 0.585714 0.6 0.614286 0.628571 0.642857 0.657143 0.671429 0.685714 0.7 0.714286 0.728571 0.742857 0.757143 0.771429 0.785714 0.8 0.814286 0.828571 0.842857 0.857143 0.871429 0.885714 0.9 0.914286 0.928571 0.942857 0.957143 0.971429 0.985714 1 1 1 1 1 1
  arc A75 (-53.0289, -4.1049) -> (-52.936, -5.1658) centre (0, 0) ccw
  spline S150 degree 5 poles (-52.936, -5.1658) (-52.9227, -5.1702) (-52.8961, -5.179) (-52.8561, -5.1921) (-52.8028, -5.2095) (-52.7362, -5.231) (-52.6695, -5.2522) (-52.6028, -5.2732) (-52.5361, -5.2939) (-52.4694, -5.3144) (-52.4027, -5.3347) (-52.3359, -5.3547) (-52.2692, -5.3744) (-52.2024, -5.3939) (-52.1356, -5.4132) (-52.0688, -5.4322) (-52.002, -5.451) (-51.9351, -5.4695) (-51.8683, -5.4877) (-51.8014, -5.5057) (-51.7346, -5.5234) (-51.6677, -5.5409) (-51.6008, -5.558) (-51.5339, -5.575) (-51.467, -5.5916) (-51.4, -5.608) (-51.3331, -5.6241) (-51.2662, -5.6399) (-51.1992, -5.6554) (-51.1323, -5.6707) (-51.0653, -5.6857) (-50.9984, -5.7003) (-50.9314, -5.7147) (-50.8644, -5.7288) (-50.7974, -5.7426) (-50.7304, -5.7561) (-50.6635, -5.7693) (-50.5965, -5.7822) (-50.5295, -5.7947) (-50.4625, -5.807) (-50.3955, -5.8189) (-50.3285, -5.8305) (-50.2615, -5.8418) (-50.2043, -5.8512) (-50.1604, -5.8581) (-50.1299, -5.8629) (-50.1128, -5.8656) (-50.1091, -5.8661) knots -1 -1 -1 -1 -1 -1 -0.985714 -0.971429 -0.957143 -0.942857 -0.928571 -0.914286 -0.9 -0.885714 -0.871429 -0.857143 -0.842857 -0.828571 -0.814286 -0.8 -0.785714 -0.771429 -0.757143 -0.742857 -0.728571 -0.714286 -0.7 -0.685714 -0.671429 -0.657143 -0.642857 -0.628571 -0.614286 -0.6 -0.585714 -0.571429 -0.557143 -0.542857 -0.528571 -0.514286 -0.5 -0.485714 -0.471429 -0.457143 -0.442857 -0.428571 -0.414286 -0.4 -0.396066 -0.396066 -0.396066 -0.396066 -0.396066 -0.396066
  spline S151 degree 3 poles (-49.6893, -6.2974) (-49.6975, -6.2328) (-49.7183, -6.1704) (-49.7824, -6.0571) (-49.8253, -6.0073) (-49.9102, -5.9407) (-49.9471, -5.9186) (-50.0256, -5.8846) (-50.0668, -5.8726) (-50.1091, -5.8661) knots 0 0 0 0 0.019532 0.019532 0.039064 0.039064 0.051902 0.051902 0.06474 0.06474 0.06474 0.06474
  arc A76 (-49.6893, -6.2974) -> (-49.6261, -6.7777) centre (0, 0) ccw
  spline S152 degree 3 poles (-49.92, -7.303) (-49.8604, -7.2767) (-49.8065, -7.2391) (-49.7162, -7.1453) (-49.6806, -7.09) (-49.6409, -6.9897) (-49.6303, -6.9481) (-49.62, -6.8631) (-49.6203, -6.8201) (-49.6261, -6.7777) knots 0 0 0 0 0.019532 0.019532 0.039064 0.039064 0.051902 0.051902 0.06474 0.06474 0.06474 0.06474
  spline S153 degree 5 poles (-49.92, -7.303) (-49.9234, -7.3045) (-49.9392, -7.3114) (-49.9674, -7.3239) (-50.008, -7.342) (-50.0609, -7.3659) (-50.1227, -7.3941) (-50.1844, -7.4227) (-50.246, -7.4515) (-50.3075, -7.4807) (-50.369, -7.5102) (-50.4303, -7.5399) (-50.4916, -7.57) (-50.5528, -7.6004) (-50.614, -7.6311) (-50.675, -7.662) (-50.736, -7.6932) (-50.7969, -7.7247) (-50.8577, -7.7565) (-50.9184, -7.7886) (-50.979, -7.8209) (-51.0396, -7.8535) (-51.1001, -7.8864) (-51.1605, -7.9196) (-51.2208, -7.9529) (-51.2811, -7.9866) (-51.3412, -8.0205) (-51.4013, -8.0547) (-51.4613, -8.0891) (-51.5212, -8.1238) (-51.5811, -8.1587) (-51.6409, -8.1939) (-51.7006, -8.2293) (-51.7602, -8.2649) (-51.8197, -8.3008) (-51.8791, -8.337) (-51.9385, -8.3733) (-51.9978, -8.4099) (-52.057, -8.4468) (-52.1162, -8.4838) (-52.1752, -8.5211) (-52.2342, -8.5587) (-52.2931, -8.5964) (-52.3519, -8.6344) (-52.3989, -8.665) (-52.4341, -8.688) (-52.4576, -8.7034) (-52.4693, -8.7111) knots 0.396066 0.396066 0.396066 0.396066 0.396066 0.396066 0.4 0.414286 0.428571 0.442857 0.457143 0.471429 0.485714 0.5 0.514286 0.528571 0.542857 0.557143 0.571429 0.585714 0.6 0.614286 0.628571 0.642857 0.657143 0.671429 0.685714 0.7 0.714286 0.728571 0.742857 0.757143 0.771429 0.785714 0.8 0.814286 0.828571 0.842857 0.857143 0.871429 0.885714 0.9 0.914286 0.928571 0.942857 0.957143 0.971429 0.985714 1 1 1 1 1 1
  arc A77 (-52.4693, -8.7111) -> (-52.2844, -9.7598) centre (0, 0) ccw
  spline S154 degree 5 poles (-52.2844, -9.7598) (-52.2707, -9.7631) (-52.2434, -9.7695) (-52.2025, -9.7791) (-52.1478, -9.7917) (-52.0796, -9.8073) (-52.0113, -9.8226) (-51.9431, -9.8377) (-51.8748, -9.8526) (-51.8066, -9.8672) (-51.7383, -9.8816) (-51.6701, -9.8957) (-51.6019, -9.9095) (-51.5336, -9.9232) (-51.4654, -9.9365) (-51.3972, -9.9496) (-51.329, -9.9625) (-51.2608, -9.9751) (-51.1926, -9.9874) (-51.1245, -9.9995) (-51.0563, -10.0114) (-50.9881, -10.0229) (-50.92, -10.0342) (-50.8519, -10.0452) (-50.7838, -10.056) (-50.7157, -10.0665) (-50.6476, -10.0767) (-50.5795, -10.0866) (-50.5115, -10.0962) (-50.4435, -10.1056) (-50.3755, -10.1147) (-50.3075, -10.1235) (-50.2395, -10.132) (-50.1715, -10.1402) (-50.1036, -10.1481) (-50.0357, -10.1557) (-49.9678, -10.163) (-49.9, -10.17) (-49.8322, -10.1766) (-49.7644, -10.183) (-49.6966, -10.189) (-49.6288, -10.1948) (-49.5611, -10.2002) (-49.5033, -10.2045) (-49.4589, -10.2076) (-49.4282, -10.2097) (-49.4109, -10.2109) (-49.4072, -10.2111) knots -1 -1 -1 -1 -1 -1 -0.985714 -0.971429 -0.957143 -0.942857 -0.928571 -0.914286 -0.9 -0.885714 -0.871429 -0.857143 -0.842857 -0.828571 -0.814286 -0.8 -0.785714 -0.771429 -0.757143 -0.742857 -0.728571 -0.714286 -0.7 -0.685714 -0.671429 -0.657143 -0.642857 -0.628571 -0.614286 -0.6 -0.585714 -0.571429 -0.557143 -0.542857 -0.528571 -0.514286 -0.5 -0.485714 -0.471429 -0.457143 -0.442857 -0.428571 -0.414286 -0.4 -0.396066 -0.396066 -0.396066 -0.396066 -0.396066 -0.396066
  spline S155 degree 3 poles (-48.9514, -10.6042) (-48.9652, -10.5405) (-48.9913, -10.4802) (-49.0651, -10.3729) (-49.1121, -10.327) (-49.2025, -10.268) (-49.2411, -10.2493) (-49.3223, -10.2222) (-49.3645, -10.2139) (-49.4072, -10.2111) knots 0 0 0 0 0.019532 0.019532 0.039064 0.039064 0.051902 0.051902 0.06474 0.06474 0.06474 0.06474
  arc A78 (-48.9514, -10.6042) -> (-48.8466, -11.0771) centre (0, 0) ccw
  spline S156 degree 3 poles (-49.0935, -11.626) (-49.0365, -11.5946) (-48.986, -11.5525) (-48.9042, -11.4512) (-48.8736, -11.393) (-48.8428, -11.2896) (-48.8359, -11.2472) (-48.833, -11.1616) (-48.8371, -11.1189) (-48.8466, -11.0771) knots 0 0 0 0 0.019532 0.019532 0.039064 0.039064 0.051902 0.051902 0.06474 0.06474 0.06474 0.06474
  spline S157 degree 5 poles (-49.0935, -11.626) (-49.0968, -11.6278) (-49.1119, -11.6361) (-49.139, -11.651) (-49.1778, -11.6726) (-49.2284, -11.701) (-49.2875, -11.7345) (-49.3465, -11.7683) (-49.4053, -11.8024) (-49.4641, -11.8368) (-49.5228, -11.8715) (-49.5813, -11.9065) (-49.6397, -11.9419) (-49.6981, -11.9774) (-49.7563, -12.0133) (-49.8144, -12.0495) (-49.8724, -12.0859) (-49.9303, -12.1226) (-49.9881, -12.1596) (-50.0458, -12.1968) (-50.1034, -12.2343) (-50.1609, -12.272) (-50.2183, -12.3101) (-50.2756, -12.3483) (-50.3328, -12.3869) (-50.3898, -12.4257) (-50.4468, -12.4647) (-50.5037, -12.504) (-50.5605, -12.5435) (-50.6172, -12.5832) (-50.6737, -12.6232) (-50.7302, -12.6635) (-50.7866, -12.704) (-50.8429, -12.7447) (-50.899, -12.7856) (-50.9551, -12.8268) (-51.0111, -12.8682) (-51.067, -12.9098) (-51.1228, -12.9517) (-51.1784, -12.9938) (-51.234, -13.0361) (-51.2895, -13.0786) (-51.3449, -13.1213) (-51.4002, -13.1643) (-51.4443, -13.1988) (-51.4774, -13.2248) (-51.4994, -13.2422) (-51.5104, -13.2509) knots 0.396066 0.396066 0.396066 0.396066 0.396066 0.396066 0.4 0.414286 0.428571 0.442857 0.457143 0.471429 0.485714 0.5 0.514286 0.528571 0.542857 0.557143 0.571429 0.585714 0.6 0.614286 0.628571 0.642857 0.657143 0.671429 0.685714 0.7 0.714286 0.728571 0.742857 0.757143 0.771429 0.785714 0.8 0.814286 0.828571 0.842857 0.857143 0.871429 0.885714 0.9 0.914286 0.928571 0.942857 0.957143 0.971429 0.985714 1 1 1 1 1 1
  arc A79 (-51.5104, -13.2509) -> (-51.2348, -14.2796) centre (0, 0) ccw
  spline S158 degree 5 poles (-51.2348, -14.2796) (-51.2209, -14.2816) (-51.1931, -14.2856) (-51.1515, -14.2916) (-51.096, -14.2995) (-51.0266, -14.309) (-50.9573, -14.3183) (-50.888, -14.3274) (-50.8187, -14.3363) (-50.7494, -14.3449) (-50.6802, -14.3532) (-50.611, -14.3614) (-50.5418, -14.3692) (-50.4727, -14.3768) (-50.4035, -14.3842) (-50.3345, -14.3913) (-50.2654, -14.3982) (-50.1964, -14.4048) (-50.1274, -14.4112) (-50.0584, -14.4173) (-49.9895, -14.4231) (-49.9206, -14.4287) (-49.8517, -14.434) (-49.7829, -14.439) (-49.7141, -14.4438) (-49.6453, -14.4483) (-49.5766, -14.4525) (-49.508, -14.4565) (-49.4393, -14.4602) (-49.3708, -14.4636) (-49.3022, -14.4667) (-49.2337, -14.4695) (-49.1653, -14.4721) (-49.0969, -14.4743) (-49.0285, -14.4763) (-48.9602, -14.4779) (-48.8919, -14.4793) (-48.8237, -14.4803) (-48.7556, -14.4811) (-48.6875, -14.4815) (-48.6194, -14.4816) (-48.5515, -14.4814) (-48.4835, -14.4809) (-48.4255, -14.4801) (-48.3811, -14.4794) (-48.3502, -14.4788) (-48.333, -14.4784) (-48.3292, -14.4784) knots -1 -1 -1 -1 -1 -1 -0.985714 -0.971429 -0.957143 -0.942857 -0.928571 -0.914286 -0.9 -0.885714 -0.871429 -0.857143 -0.842857 -0.828571 -0.814286 -0.8 -0.785714 -0.771429 -0.757143 -0.742857 -0.728571 -0.714286 -0.7 -0.685714 -0.671429 -0.657143 -0.642857 -0.628571 -0.614286 -0.6 -0.585714 -0.571429 -0.557143 -0.542857 -0.528571 -0.514286 -0.5 -0.485714 -0.471429 -0.457143 -0.442857 -0.428571 -0.414286 -0.4 -0.396066 -0.396066 -0.396066 -0.396066 -0.396066 -0.396066
  spline S159 degree 3 poles (-47.8409, -14.8302) (-47.8602, -14.768) (-47.8914, -14.7102) (-47.9743, -14.6098) (-48.0252, -14.5681) (-48.1203, -14.5172) (-48.1605, -14.5019) (-48.2437, -14.482) (-48.2864, -14.4774) (-48.3292, -14.4784) knots 0 0 0 0 0.019532 0.019532 0.039064 0.039064 0.051902 0.051902 0.06474 0.06474 0.06474 0.06474
  arc A80 (-47.8409, -14.8302) -> (-47.6952, -15.2922) centre (0, 0) ccw
  spline S160 degree 3 poles (-47.8934, -15.8605) (-47.8393, -15.8243) (-47.7928, -15.7779) (-47.7201, -15.6699) (-47.6947, -15.6093) (-47.673, -15.5036) (-47.6698, -15.4607) (-47.6744, -15.3752) (-47.6822, -15.333) (-47.6952, -15.2922) knots 0 0 0 0 0.019532 0.019532 0.039064 0.039064 0.051902 0.051902 0.06474 0.06474 0.06474 0.06474